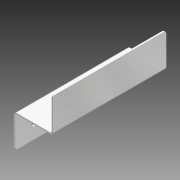
# Autodesk Inventor part: FE-120-010 Tube Holder
Saved by Autodesk Inventor 2021 (Build 250183000, 183)
## iProperties
Created: 2021-01-12
Part Number: FE-120-010 Tube Holder
Material: Aluminum 6061
Document SubType Name: Sheet Metal
Density: 2.7 g/cm^3
Sheet Metal Rule: Default
Appearance: Aluminum - Dark
Autodesk Inventor part; units mm, degrees
ref_plane "YZ Plane" through (0, 0, 0) normal (1, 0, 0) x (0, 1, 0)
ref_plane "XZ Plane" through (0, 0, 0) normal (0, 1, 0) x (-1, 0, 0)
ref_plane "XY Plane" through (0, 0, 0) normal (0, 0, 1) x (1, 0, 0)
sketch "Sketch1" plane through (0, 0, 0) normal (0, 0, 1) x (1, 0, 0)
  line L0 (0, 0) -> (-50.8, 0)
  line L1 (-50.8, 0) -> (-50.8, -44.45)
  line L2 (0, 0) -> (0, 44.45)
  dimension "d0" = 50.8
  dimension "d1" = 44.45
  dimension "d2" = 44.45
  measures "d0" distance of L0.start L0.end
  measures "d1" distance of L0.end L1.end
  measures "d2" distance of L0.start L2.end
contour flange "Contour Flange1" sketch "Sketch1" thickness 2.032 bend radius 2.032 width 152.4 along (0, 0, 1) mid plane no both sides no wall seen from (-50.8, -22.225, 0) lies toward (1, 0, 0) curves L1 L0 L2
bend "Bend1"
corner "Corner1"
sketch "Sketch2" plane through (-50.8, -44.45, 0) normal (-1, 0, 0) x (0, 0, 1)
  circle A0 centre (127, 19.05) radius 3.3655
  circle A1 centre (25.4, 19.05) radius 3.3655
  line L0 (152.4, 0) -> (0, 0) projected
  line L1 (152.4, 40.386) -> (152.4, 0) projected
  line L2 (0, 0) -> (0, 40.386) projected
  point P0 (0, 44.45)
  dimension "d14" = 6.731
  dimension "d15" = 19.05
  dimension "d16" = 25.4
  dimension "d17" = 25.4
  constraints: 2 centre point, 1 equal radius, 1 horizontal alignment
  measures "d14" diameter of A0
  measures "d15" distance from line of L0 A0.centre
  measures "d16" distance from line of L1 A0.centre
  measures "d17" distance from line of A1.centre L2
extrude "Cut1" cut sketch "Sketch2" against normal blind 2.032
fillet "Corner Round1" radius 3.175 4 edges at (1.016, 44.45, 0) (-49.784, -44.45, 152.4) (1.016, 44.45, 152.4) (-49.784, -44.45, 0)
equation "\"d17\" = d16"
equation "\"d18\" = Thickness"
equation "\"d3\" = Thickness"
equation "\"d4\" = BendReliefWidth"
equation "\"d5\" = BendReliefDepth"
equation "\"d6\" = MinimumRemnant"
equation "\"d7\" = TransitionRadius"
equation "\"d9\" = BendRadius"
equation "\"d11\" = CornerReliefSize"
equation "\"d12\" = GapSize"
equation "\"d13\" = JacobiRadiusSize"
equation "\"BendRadius\" = Thickness"
equation "\"BendReliefWidth\" = Thickness"
equation "\"BendReliefDepth\" = 0.5 * Thickness"
equation "\"CornerReliefSize\" = 4 * Thickness"
equation "\"MinimumRemnant\" = 2 * Thickness"
equation "\"TransitionRadius\" = BendRadius"
equation "\"JacobiRadiusSize\" = Thickness"
equation "\"GapSize\" = Thickness"
equation "\"Thickness\" = 2.032"
body "Solid1"
